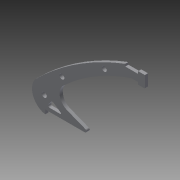
# Autodesk Inventor part: Side_Part
Saved by Autodesk Inventor 2014 SP1 (Build 180222100, 222)
## iProperties
Created: 2014-07-27
Part Number: Side_Part
Material: Generic
Document SubType Name: Modeling
Designer: Ryan
Density: 1 g/cm^3
Appearance: Default
Author: Ryan
Autodesk Inventor part; units mm, degrees
ref_plane "YZ Plane" through (0, 0, 0) normal (1, 0, 0) x (0, 1, 0)
ref_plane "XZ Plane" through (0, 0, 0) normal (0, 1, 0) x (-1, 0, 0)
ref_plane "XY Plane" through (0, 0, 0) normal (0, 0, 1) x (1, 0, 0)
sketch "Side Part" plane through (0, 0, 0) normal (0, 0, 1) x (1, 0, 0)
  arc A0 (59.2149, 53.2214) -> (1.9677, 16.0747) centre (117.7132, -99.6165) ccw
  arc A1 (63.2649, 47.3171) -> (19.3751, 21.046) centre (99.8299, -63.5681) ccw
  arc A2 (19.3751, 21.046) -> (22.0544, 9.2781) centre (24.9814, 16.1335) ccw
  arc A3 (1.9677, 16.0747) -> (8.356, 0) centre (10.2097, 10.0435) ccw
  circle A4 centre (18.9507, 26.1162) radius 1.6
  circle A5 centre (45.9082, 43.8146) radius 1.6
  line L0 (8.356, 0) -> (8.356, 2.7)
  line L1 (59.2149, 53.2214) -> (59.2149, 51.7214)
  line L2 (59.2149, 51.7214) -> (67.3149, 51.7214)
  line L3 (67.3149, 51.7214) -> (67.3149, 53.2214)
  line L4 (71.631, 46.0171) -> (71.631, 53.0214)
  line L5 (67.3149, 53.2214) -> (71.431, 53.2214)
  arc A6 (71.631, 53.0214) -> (71.431, 53.2214) centre (71.431, 53.0214) ccw
  arc A7 (22.0544, 9.2781) -> (22.0677, 9.2723) centre (22.1405, 9.4586) ccw
  circle A8 centre (7.756, 10.482) radius 1.6
  line L6 (12.2179, 8.9259) -> (10.405, 6.6138)
  arc A9 (10.405, 6.6138) -> (11.1919, 4.9967) centre (11.1919, 5.9967) ccw
  line L7 (11.1919, 4.9967) -> (17.8503, 4.9967)
  line L8 (18.1389, 5.9051) -> (13.582, 9.1255)
  arc A10 (17.8503, 4.9967) -> (18.1389, 5.9051) centre (17.8503, 5.4967) ccw
  arc A11 (13.582, 9.1255) -> (12.2179, 8.9259) centre (13.0048, 8.3088) ccw
  line L9 (8.356, 2.7) -> (33.5768, 2.7)
  arc A12 (33.5768, 2.7) -> (33.9408, 4.6314) centre (33.5768, 3.7) ccw
  line L10 (33.9408, 4.6314) -> (22.0677, 9.2723)
  line L11 (67.3149, 45.8171) -> (67.3149, 47.3171)
  line L12 (67.3149, 45.8171) -> (71.431, 45.8171)
  arc A13 (71.431, 45.8171) -> (71.631, 46.0171) centre (71.431, 46.0171) ccw
  line L13 (63.2649, 47.3171) -> (67.3149, 47.3171)
  point P0 (38.6259, 23.714)
sketch "Sketch1" plane through (0, 0, 0) normal (0, 0, 1) x (1, 0, 0)
  circle A0 centre (45.9082, 43.8146) radius 1.6
  circle A1 centre (18.9507, 26.1162) radius 1.6
  circle A2 centre (7.756, 10.482) radius 1.6
  arc A3 (10.405, 6.6138) -> (11.1919, 4.9967) centre (11.1919, 5.9967) ccw
  arc A4 (13.582, 9.1255) -> (12.2179, 8.9259) centre (13.0048, 8.3088) ccw
  arc A5 (17.8503, 4.9967) -> (18.1389, 5.9051) centre (17.8503, 5.4967) ccw
  arc A6 (20.4302, 22.0369) -> (22.4669, 9.1163) centre (24.9814, 16.1335) ccw
  arc A7 (33.5768, 2.7) -> (33.9408, 4.6314) centre (33.5768, 3.7) ccw
  arc A8 (4.3433, 18.4037) -> (8.356, 0) centre (10.2097, 10.0435) ccw
  line L0 (8.356, 0) -> (8.356, 2.7)
  line L1 (8.356, 2.7) -> (33.5768, 2.7)
  line L2 (33.9408, 4.6314) -> (22.4669, 9.1163)
  line L3 (18.1389, 5.9051) -> (13.582, 9.1255)
  line L4 (11.1919, 4.9967) -> (17.8503, 4.9967)
  line L5 (12.2179, 8.9259) -> (10.405, 6.6138)
  arc A9 (59.2149, 53.2214) -> (1.9677, 16.0747) centre (117.7132, -99.6165) ccw
  arc A10 (63.2649, 47.3171) -> (19.3751, 21.046) centre (99.8299, -63.5681) ccw
  line L6 (59.2149, 53.2214) -> (59.2149, 51.7214)
  line L7 (59.2149, 51.7214) -> (67.3149, 51.7214)
  line L8 (67.3149, 51.7214) -> (67.3149, 53.2214)
  arc A11 (71.631, 53.0214) -> (71.431, 53.2214) centre (71.431, 53.0214) ccw
  arc A12 (71.431, 45.8171) -> (71.631, 46.0171) centre (71.431, 46.0171) ccw
  line L9 (67.3149, 53.2214) -> (71.431, 53.2214)
  line L10 (71.631, 53.0214) -> (71.631, 46.0171)
  line L11 (71.431, 45.8171) -> (67.3149, 45.8171)
  line L12 (67.3149, 45.8171) -> (67.3149, 47.3171)
  line L13 (67.3149, 47.3171) -> (63.2649, 47.3171)
  arc A13 (59.2149, 53.2214) -> (1.9677, 16.0747) centre (117.7132, -99.6165) ccw
  arc A14 (63.2649, 47.3171) -> (19.3751, 21.046) centre (99.8299, -63.5681) ccw
  arc A15 (19.3751, 21.046) -> (22.0544, 9.2781) centre (24.9814, 16.1335) ccw
  arc A16 (1.9677, 16.0747) -> (8.356, 0) centre (10.2097, 10.0435) ccw
  circle A17 centre (18.9507, 26.1162) radius 1.6
  circle A18 centre (45.9082, 43.8146) radius 1.6
  line L14 (8.356, 0) -> (8.356, 2.7)
  line L15 (59.2149, 53.2214) -> (59.2149, 51.7214)
  line L16 (59.2149, 51.7214) -> (67.3149, 51.7214)
  line L17 (67.3149, 51.7214) -> (67.3149, 53.2214)
  line L18 (71.631, 46.0171) -> (71.631, 53.0214)
  line L19 (67.3149, 53.2214) -> (71.431, 53.2214)
  arc A19 (71.631, 53.0214) -> (71.431, 53.2214) centre (71.431, 53.0214) ccw
  arc A20 (22.0544, 9.2781) -> (22.0677, 9.2723) centre (22.1405, 9.4586) ccw
  circle A21 centre (7.756, 10.482) radius 1.6
  line L20 (12.2179, 8.9259) -> (10.405, 6.6138)
  arc A22 (10.405, 6.6138) -> (11.1919, 4.9967) centre (11.1919, 5.9967) ccw
  line L21 (11.1919, 4.9967) -> (17.8503, 4.9967)
  line L22 (18.1389, 5.9051) -> (13.582, 9.1255)
  arc A23 (17.8503, 4.9967) -> (18.1389, 5.9051) centre (17.8503, 5.4967) ccw
  arc A24 (13.582, 9.1255) -> (12.2179, 8.9259) centre (13.0048, 8.3088) ccw
  line L23 (8.356, 2.7) -> (33.5768, 2.7)
  arc A25 (33.5768, 2.7) -> (33.9408, 4.6314) centre (33.5768, 3.7) ccw
  line L24 (33.9408, 4.6314) -> (22.0677, 9.2723)
  line L25 (67.3149, 45.8171) -> (67.3149, 47.3171)
  line L26 (67.3149, 45.8171) -> (71.431, 45.8171)
  arc A26 (71.431, 45.8171) -> (71.631, 46.0171) centre (71.431, 46.0171) ccw
  line L27 (63.2649, 47.3171) -> (67.3149, 47.3171)
  point P0 (0, 0)
  constraints: 28 end point, 24 point on circle, 13 centre point, 12 tangent, 9 horizontal, 6 vertical, 1 perpendicular, 54 other
extrude "Extrusion1" add sketch "Sketch1" along normal blind 2 contours A6 L2 A7 L1 L0 A8 A9 L6 L7 L8 L9 A11 L10 A12 L11 L12 L13 A10
body "Solid1"
